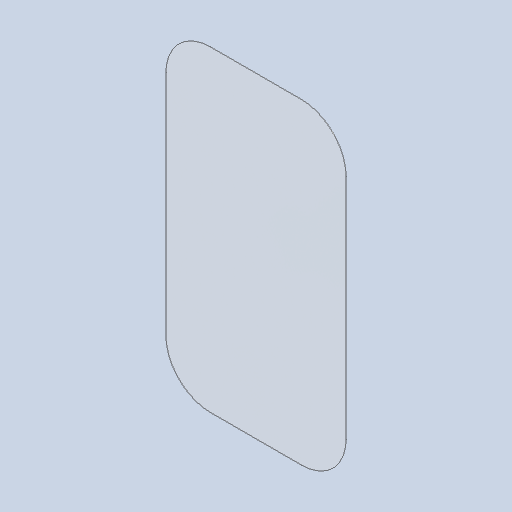
# Autodesk Inventor part: PLatico
Saved by Autodesk Inventor 2023 (Build 270158000, 158)
## iProperties
Created: 2022-11-28
Part Number: PLatico
Material: Plastic, Transparent
Document SubType Name: Modeling
Designer: David
Density: 1.188 g/cm^3
Appearance: Transparent - Clear
Author: David
Autodesk Inventor part; units mm, degrees
ref_plane "YZ Plane" through (0, 0, 0) normal (1, 0, 0) x (0, 1, 0)
ref_plane "XZ Plane" through (0, 0, 0) normal (0, 1, 0) x (-1, 0, 0)
ref_plane "XY Plane" through (0, 0, 0) normal (0, 0, 1) x (1, 0, 0)
sketch "Sketch1" plane through (0, 0, 0) normal (0, 0, 1) x (1, 0, 0)
  line L0 (0, -500) -> (900, -500)
  line L1 (900, -500) -> (900, 850)
  line L2 (900, 850) -> (0, 850)
  line L3 (0, 850) -> (0, -500)
  line L4 (0, -500) -> (900, 850) construction
  line L5 (900, -500) -> (0, 850) construction
  line L6 (300, 700) -> (600, 700)
  line L7 (750, 550) -> (750, -200)
  line L8 (600, -350) -> (300, -350)
  line L9 (150, -200) -> (150, 550)
  arc A0 (750, 550) -> (600, 700) centre (600, 550) ccw
  arc A1 (300, 700) -> (150, 550) centre (300, 550) ccw
  arc A2 (150, -200) -> (300, -350) centre (300, -200) ccw
  arc A3 (600, -350) -> (750, -200) centre (600, -200) ccw
  line L10 (600, 697) -> (300, 697)
  arc A4 (300, 697) -> (153, 550) centre (300, 550) ccw
  line L11 (153, 550) -> (153, -200)
  arc A5 (153, -200) -> (300, -347) centre (300, -200) ccw
  line L12 (300, -347) -> (600, -347)
  arc A6 (600, -347) -> (747, -200) centre (600, -200) ccw
  line L13 (747, -200) -> (747, 550)
  arc A7 (747, 550) -> (600, 697) centre (600, 550) ccw
  point P0 (0, 0)
  point P1 (0, 0)
  point P2 (450, 175)
  dimension "d0" = 900
  dimension "d1" = 1350
  dimension "d2" = 150
  dimension "d3" = 150
  dimension "d4" = 150
  dimension "d5" = 150
  dimension "d6" = 150
  dimension "d7" = 3
  dimension "d10" = 1044
  constraints: 28 end point, 16 point on circle, 8 centre point, 8 tangent, 6 parallel, 3 perpendicular, 2 midpoint, 1 horizontal, 10 other
  measures "d0" distance of L2.end L1.end
  measures "d1" distance of L1.end L0.end
  measures "d2" distance between parallel lines of L2 L6
  measures "d3" radius of A0
  measures "d4" radius of A1
  measures "d5" radius of A2
  measures "d6" radius of A3
  measures "d7" distance between parallel lines of L6 L10
  measures "d10" distance between parallel lines of L12 L10
extrude "Extrusion1" add sketch "Sketch1" along normal mid plane 2 contours A7 L13 A6 L12 A5 L11 A4 L10
equation "\"Space5\" = 0"
equation "\"Space6\" = 0"
equation "\"Space7\" = 0"
body "Solid1"
